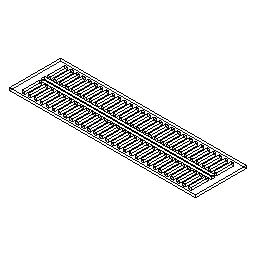
shelf small v2 (Autodesk Fusion 360 design; units mm, degrees)
Autodesk Fusion 360 part; units mm, degrees
sketch "Sketch1" plane through (0, 0, 0) normal (0, 0, 1) x (1, 0, 0)
  line L0 (109.5, -30) -> (-109.5, -30)
  line L1 (-109.5, -30) -> (-109.5, 30)
  line L2 (-109.5, 30) -> (109.5, 30)
  line L3 (109.5, 30) -> (109.5, -30)
  line L4 (109.5, -30) -> (-109.5, 30) construction
  line L5 (-109.5, -30) -> (109.5, 30) construction
  dimension "d1" = 60
  dimension "d2" = 219
  constraint horizontal L0
  constraint perpendicular L0 L1
  constraint parallel L0 L2
  constraint parallel L1 L3
  constraint coincident L4 origin
  constraint coincident L5 origin
  measures "d1" distance of L0.end L1.end
  measures "d2" distance of L1.end L2.end
extrude "Extrude1" add sketch "Sketch1" along normal blind 3
sketch "Sketch2" plane through (0, 0, 3) normal (0, 0, 1) x (-1, 0, 0)
  line L0 (-109.5, -30) -> (109.5, -30)
  line L1 (109.5, -30) -> (109.5, 30)
  line L2 (109.5, 30) -> (-109.5, 30)
  line L3 (-109.5, 30) -> (-109.5, -30)
  line L4 (-100, 2) -> (100, 2)
  line L5 (100, 2) -> (100, -2)
  line L6 (100, -2) -> (-100, -2)
  line L7 (-100, -2) -> (-100, 2)
  line L8 (-100, 2) -> (100, -2) construction
  line L9 (100, 2) -> (-100, -2) construction
  line L10 (36.5, -25) -> (33.5, -25)
  line L11 (33.5, -25) -> (33.5, -5)
  line L12 (33.5, -5) -> (36.5, -5)
  line L13 (36.5, -5) -> (36.5, -25)
  line L14 (29.5, -25) -> (26.5, -25)
  line L15 (26.5, -25) -> (26.5, -5)
  line L16 (26.5, -5) -> (29.5, -5)
  line L17 (29.5, -5) -> (29.5, -25)
  line L18 (22.5, -25) -> (19.5, -25)
  line L19 (19.5, -25) -> (19.5, -5)
  line L20 (19.5, -5) -> (22.5, -5)
  line L21 (22.5, -5) -> (22.5, -25)
  line L22 (15.5, -25) -> (12.5, -25)
  line L23 (12.5, -25) -> (12.5, -5)
  line L24 (12.5, -5) -> (15.5, -5)
  line L25 (15.5, -5) -> (15.5, -25)
  line L26 (8.5, -25) -> (5.5, -25)
  line L27 (5.5, -25) -> (5.5, -5)
  line L28 (5.5, -5) -> (8.5, -5)
  line L29 (8.5, -5) -> (8.5, -25)
  line L30 (1.5, -25) -> (-1.5, -25)
  line L31 (-1.5, -25) -> (-1.5, -5)
  line L32 (-1.5, -5) -> (1.5, -5)
  line L33 (1.5, -5) -> (1.5, -25)
  line L34 (-5.5, -25) -> (-8.5, -25)
  line L35 (-8.5, -25) -> (-8.5, -5)
  line L36 (-8.5, -5) -> (-5.5, -5)
  line L37 (-5.5, -5) -> (-5.5, -25)
  line L38 (-12.5, -25) -> (-15.5, -25)
  line L39 (-15.5, -25) -> (-15.5, -5)
  line L40 (-15.5, -5) -> (-12.5, -5)
  line L41 (-12.5, -5) -> (-12.5, -25)
  line L42 (-19.5, -25) -> (-22.5, -25)
  line L43 (-22.5, -25) -> (-22.5, -5)
  line L44 (-22.5, -5) -> (-19.5, -5)
  line L45 (-19.5, -5) -> (-19.5, -25)
  line L46 (-26.5, -25) -> (-29.5, -25)
  line L47 (-29.5, -25) -> (-29.5, -5)
  line L48 (-29.5, -5) -> (-26.5, -5)
  line L49 (-26.5, -5) -> (-26.5, -25)
  line L50 (-33.5, -25) -> (-36.5, -25)
  line L51 (-36.5, -25) -> (-36.5, -5)
  line L52 (-36.5, -5) -> (-33.5, -5)
  line L53 (-33.5, -5) -> (-33.5, -25)
  line L54 (-40.5, -25) -> (-43.5, -25)
  line L55 (-43.5, -25) -> (-43.5, -5)
  line L56 (-43.5, -5) -> (-40.5, -5)
  line L57 (-40.5, -5) -> (-40.5, -25)
  line L58 (-47.5, -25) -> (-50.5, -25)
  line L59 (-50.5, -25) -> (-50.5, -5)
  line L60 (-50.5, -5) -> (-47.5, -5)
  line L61 (-47.5, -5) -> (-47.5, -25)
  line L62 (-54.5, -25) -> (-57.5, -25)
  line L63 (-57.5, -25) -> (-57.5, -5)
  line L64 (-57.5, -5) -> (-54.5, -5)
  line L65 (-54.5, -5) -> (-54.5, -25)
  line L66 (-61.5, -25) -> (-64.5, -25)
  line L67 (-64.5, -25) -> (-64.5, -5)
  line L68 (-64.5, -5) -> (-61.5, -5)
  line L69 (-61.5, -5) -> (-61.5, -25)
  line L70 (-68.5, -25) -> (-71.5, -25)
  line L71 (-71.5, -25) -> (-71.5, -5)
  line L72 (-71.5, -5) -> (-68.5, -5)
  line L73 (-68.5, -5) -> (-68.5, -25)
  line L74 (-75.5, -5) -> (-78.5, -5)
  line L75 (-78.5, -5) -> (-78.5, -25)
  line L76 (-78.5, -25) -> (-75.5, -25)
  line L77 (-75.5, -25) -> (-75.5, -5)
  line L78 (-82.5, -5) -> (-85.5, -5)
  line L79 (-85.5, -5) -> (-85.5, -25)
  line L80 (-85.5, -25) -> (-82.5, -25)
  line L81 (-82.5, -25) -> (-82.5, -5)
  line L82 (-89.5, -5) -> (-92.5, -5)
  line L83 (-92.5, -5) -> (-92.5, -25)
  line L84 (-92.5, -25) -> (-89.5, -25)
  line L85 (-89.5, -25) -> (-89.5, -5)
  line L86 (-96.5, -5) -> (-99.5, -5)
  line L87 (-99.5, -5) -> (-99.5, -25)
  line L88 (-99.5, -25) -> (-96.5, -25)
  line L89 (-96.5, -25) -> (-96.5, -5)
  line L90 (36.5, 5) -> (33.5, 5)
  line L91 (33.5, 5) -> (33.5, 25)
  line L92 (33.5, 25) -> (36.5, 25)
  line L93 (36.5, 25) -> (36.5, 5)
  line L94 (29.5, 5) -> (26.5, 5)
  line L95 (26.5, 5) -> (26.5, 25)
  line L96 (26.5, 25) -> (29.5, 25)
  line L97 (29.5, 25) -> (29.5, 5)
  line L98 (22.5, 5) -> (19.5, 5)
  line L99 (19.5, 5) -> (19.5, 25)
  line L100 (19.5, 25) -> (22.5, 25)
  line L101 (22.5, 25) -> (22.5, 5)
  line L102 (15.5, 5) -> (12.5, 5)
  line L103 (12.5, 5) -> (12.5, 25)
  line L104 (12.5, 25) -> (15.5, 25)
  line L105 (15.5, 25) -> (15.5, 5)
  line L106 (8.5, 5) -> (5.5, 5)
  line L107 (5.5, 5) -> (5.5, 25)
  line L108 (5.5, 25) -> (8.5, 25)
  line L109 (8.5, 25) -> (8.5, 5)
  line L110 (1.5, 5) -> (-1.5, 5)
  line L111 (-1.5, 5) -> (-1.5, 25)
  line L112 (-1.5, 25) -> (1.5, 25)
  line L113 (1.5, 25) -> (1.5, 5)
  line L114 (-5.5, 5) -> (-8.5, 5)
  line L115 (-8.5, 5) -> (-8.5, 25)
  line L116 (-8.5, 25) -> (-5.5, 25)
  line L117 (-5.5, 25) -> (-5.5, 5)
  line L118 (-12.5, 5) -> (-15.5, 5)
  line L119 (-15.5, 5) -> (-15.5, 25)
  line L120 (-15.5, 25) -> (-12.5, 25)
  line L121 (-12.5, 25) -> (-12.5, 5)
  line L122 (-19.5, 5) -> (-22.5, 5)
  line L123 (-22.5, 5) -> (-22.5, 25)
  line L124 (-22.5, 25) -> (-19.5, 25)
  line L125 (-19.5, 25) -> (-19.5, 5)
  line L126 (-26.5, 5) -> (-29.5, 5)
  line L127 (-29.5, 5) -> (-29.5, 25)
  line L128 (-29.5, 25) -> (-26.5, 25)
  line L129 (-26.5, 25) -> (-26.5, 5)
  line L130 (-33.5, 5) -> (-36.5, 5)
  line L131 (-36.5, 5) -> (-36.5, 25)
  line L132 (-36.5, 25) -> (-33.5, 25)
  line L133 (-33.5, 25) -> (-33.5, 5)
  line L134 (-40.5, 5) -> (-43.5, 5)
  line L135 (-43.5, 5) -> (-43.5, 25)
  line L136 (-43.5, 25) -> (-40.5, 25)
  line L137 (-40.5, 25) -> (-40.5, 5)
  line L138 (-47.5, 5) -> (-50.5, 5)
  line L139 (-50.5, 5) -> (-50.5, 25)
  line L140 (-50.5, 25) -> (-47.5, 25)
  line L141 (-47.5, 25) -> (-47.5, 5)
  line L142 (-54.5, 5) -> (-57.5, 5)
  line L143 (-57.5, 5) -> (-57.5, 25)
  line L144 (-57.5, 25) -> (-54.5, 25)
  line L145 (-54.5, 25) -> (-54.5, 5)
  line L146 (-61.5, 5) -> (-64.5, 5)
  line L147 (-64.5, 5) -> (-64.5, 25)
  line L148 (-64.5, 25) -> (-61.5, 25)
  line L149 (-61.5, 25) -> (-61.5, 5)
  line L150 (-68.5, 5) -> (-71.5, 5)
  line L151 (-71.5, 5) -> (-71.5, 25)
  line L152 (-71.5, 25) -> (-68.5, 25)
  line L153 (-68.5, 25) -> (-68.5, 5)
  line L154 (-75.5, 5) -> (-78.5, 5)
  line L155 (-78.5, 5) -> (-78.5, 25)
  line L156 (-78.5, 25) -> (-75.5, 25)
  line L157 (-75.5, 25) -> (-75.5, 5)
  line L158 (-82.5, 5) -> (-85.5, 5)
  line L159 (-85.5, 5) -> (-85.5, 25)
  line L160 (-85.5, 25) -> (-82.5, 25)
  line L161 (-82.5, 25) -> (-82.5, 5)
  line L162 (-89.5, 5) -> (-92.5, 5)
  line L163 (-92.5, 5) -> (-92.5, 25)
  line L164 (-92.5, 25) -> (-89.5, 25)
  line L165 (-89.5, 25) -> (-89.5, 5)
  line L166 (-96.5, 5) -> (-99.5, 5)
  line L167 (-99.5, 5) -> (-99.5, 25)
  line L168 (-99.5, 25) -> (-96.5, 25)
  line L169 (-96.5, 25) -> (-96.5, 5)
  dimension "d5" = 200
  dimension "d6" = 4
  dimension "d7" = 3
  dimension "d8" = 3
  dimension "d9" = 3
  dimension "d10" = 3
  dimension "d11" = 3
  dimension "d12" = 3
  dimension "d13" = 3
  dimension "d14" = 4
  dimension "d15" = 4
  dimension "d16" = 4
  dimension "d17" = 4
  dimension "d18" = 4
  dimension "d19" = 4
  dimension "d20" = 4
  dimension "d21" = 4
  dimension "d22" = 4
  dimension "d23" = 4
  dimension "d24" = 4
  dimension "d25" = 4
  dimension "d26" = 4
  dimension "d27" = 4
  dimension "d28" = 4
  dimension "d29" = 4
  dimension "d30" = 4
  dimension "d31" = 4
  dimension "d32" = 4
  dimension "d33" = 3
  dimension "d34" = 3
  dimension "d35" = 3
  dimension "d36" = 3
  dimension "d37" = 3
  dimension "d38" = 3
  dimension "d39" = 3
  dimension "d40" = 3
  dimension "d42" = 3
  dimension "d43" = 3
  dimension "d44" = 3
  dimension "d45" = 3
  dimension "d46" = 3
  dimension "d47" = 3
  dimension "d48" = 3
  dimension "d49" = 3
  dimension "d50" = 3
  dimension "d51" = 3
  dimension "d52" = 3
  dimension "d53" = 3
  dimension "d54" = 3
  dimension "d55" = 3
  dimension "d56" = 3
  dimension "d57" = 3
  dimension "d58" = 3
  dimension "d59" = 3
  dimension "d60" = 3
  dimension "d61" = 3
  dimension "d62" = 3
  dimension "d63" = 3
  dimension "d64" = 3
  dimension "d65" = 3
  dimension "d66" = 3
  dimension "d67" = 4
  dimension "d68" = 4
  dimension "d69" = 4
  dimension "d70" = 4
  dimension "d71" = 4
  dimension "d72" = 4
  dimension "d73" = 4
  dimension "d74" = 4
  dimension "d75" = 4
  dimension "d76" = 4
  dimension "d77" = 4
  dimension "d78" = 4
  dimension "d79" = 4
  dimension "d80" = 4
  dimension "d81" = 4
  dimension "d82" = 4
  dimension "d83" = 4
  dimension "d84" = 4
  dimension "d85" = 4
  dimension "d86" = 10
  dimension "d87" = 10
  constraint horizontal L4
  constraint perpendicular L4 L5
  constraint parallel L4 L6
  constraint parallel L5 L7
  constraint coincident L8 origin
  constraint coincident L9 origin
  constraint horizontal L10
  constraint vertical L11
  constraint horizontal L12
  constraint vertical L13
  constraint horizontal L14
  constraint vertical L15
  constraint horizontal L16
  constraint vertical L17
  constraint horizontal L18
  constraint vertical L19
  constraint horizontal L20
  constraint vertical L21
  constraint horizontal L22
  constraint vertical L23
  constraint horizontal L24
  constraint vertical L25
  constraint horizontal L26
  constraint vertical L27
  constraint horizontal L28
  constraint vertical L29
  constraint horizontal L30
  constraint vertical L31
  constraint horizontal L32
  constraint vertical L33
  constraint horizontal L34
  constraint vertical L35
  constraint horizontal L36
  constraint vertical L37
  constraint horizontal L38
  constraint vertical L39
  constraint horizontal L40
  constraint vertical L41
  constraint horizontal L42
  constraint vertical L43
  constraint horizontal L44
  constraint vertical L45
  constraint horizontal L46
  constraint vertical L47
  constraint horizontal L48
  constraint vertical L49
  constraint horizontal L50
  constraint vertical L51
  constraint horizontal L52
  constraint vertical L53
  constraint horizontal L54
  constraint vertical L55
  constraint horizontal L56
  constraint vertical L57
  constraint horizontal L58
  constraint vertical L59
  constraint horizontal L60
  constraint vertical L61
  constraint horizontal L62
  constraint vertical L63
  constraint horizontal L64
  constraint vertical L65
  constraint horizontal L66
  constraint vertical L67
  constraint horizontal L68
  constraint vertical L69
  constraint horizontal L70
  constraint vertical L71
  constraint horizontal L72
  constraint vertical L73
  constraint horizontal L74
  constraint vertical L75
  constraint horizontal L76
  constraint vertical L77
  constraint horizontal L78
  constraint vertical L79
  constraint horizontal L80
  constraint vertical L81
  constraint horizontal L82
  constraint vertical L83
  constraint horizontal L84
  constraint vertical L85
  constraint horizontal L86
  constraint vertical L87
  constraint horizontal L88
  constraint vertical L89
  constraint horizontal L90
  constraint vertical L91
  constraint horizontal L92
  constraint vertical L93
  constraint horizontal L94
  constraint vertical L95
  constraint horizontal L96
  constraint vertical L97
  constraint horizontal L98
  constraint vertical L99
  constraint horizontal L100
  constraint vertical L101
  constraint horizontal L102
  constraint vertical L103
  constraint horizontal L104
  constraint vertical L105
  constraint horizontal L106
  constraint vertical L107
  constraint horizontal L108
  constraint vertical L109
  constraint horizontal L110
  constraint vertical L111
  constraint horizontal L112
  constraint vertical L113
  constraint horizontal L114
  constraint vertical L115
  constraint horizontal L116
  constraint vertical L117
  constraint horizontal L118
  constraint vertical L119
  constraint horizontal L120
  constraint vertical L121
  constraint horizontal L122
  constraint vertical L123
  constraint horizontal L124
  constraint vertical L125
  constraint horizontal L126
  constraint vertical L127
  constraint horizontal L128
  constraint vertical L129
  constraint horizontal L130
  constraint vertical L131
  constraint horizontal L132
  constraint vertical L133
  constraint horizontal L134
  constraint vertical L135
  constraint horizontal L136
  constraint vertical L137
  constraint horizontal L138
  constraint vertical L139
  constraint horizontal L140
  constraint vertical L141
  constraint horizontal L142
  constraint vertical L143
  constraint horizontal L144
  constraint vertical L145
  constraint horizontal L146
  constraint vertical L147
  constraint horizontal L148
  constraint vertical L149
  constraint horizontal L150
  constraint vertical L151
  constraint horizontal L152
  constraint vertical L153
  constraint horizontal L154
  constraint vertical L155
  constraint horizontal L156
  constraint vertical L157
  constraint horizontal L158
  constraint vertical L159
  constraint horizontal L160
  constraint vertical L161
  constraint horizontal L162
  constraint vertical L163
  constraint horizontal L164
  constraint vertical L165
  constraint horizontal L166
  constraint vertical L167
  constraint horizontal L168
  constraint vertical L169
  measures "d5" distance of L5.end L6.end
  measures "d6" distance of L4.end L5.end
  measures "d7" distance of L10.start L10.end
  measures "d8" distance of L14.start L14.end
  measures "d9" distance of L18.start L18.end
  measures "d10" distance of L22.start L22.end
  measures "d11" distance of L26.start L26.end
  measures "d12" distance of L30.start L30.end
  measures "d13" distance of L34.start L34.end
  measures "d14" distance of L11 L17
  measures "d15" distance of L15 L21
  measures "d16" distance of L19 L25
  measures "d17" distance of L23 L29
  measures "d18" distance of L27 L33
  measures "d19" distance of L31 L37
  measures "d20" distance of L35 L41
  measures "d21" distance of L39 L45
  measures "d22" distance of L43 L49
  measures "d23" distance of L47 L53
  measures "d24" distance of L51 L57
  measures "d25" distance of L55 L61
  measures "d26" distance of L59 L65
  measures "d27" distance of L63 L69
  measures "d28" distance of L67 L73
  measures "d29" distance of L71 L77
  measures "d30" distance of L75 L81
  measures "d31" distance of L79 L85
  measures "d32" distance of L83 L89
  measures "d33" distance of L38.start L38.end
  measures "d34" distance of L42.start L42.end
  measures "d35" distance of L46.start L46.end
  measures "d36" distance of L50.start L50.end
  measures "d37" distance of L54.start L54.end
  measures "d38" distance of L58.start L58.end
  measures "d39" distance of L62.start L62.end
  measures "d40" distance of L66.start L66.end
  measures "d42" distance of L70.start L70.end
  measures "d43" distance of L75.end L76.end
  measures "d44" distance of L79.end L80.end
  measures "d45" distance of L83.end L84.end
  measures "d46" distance of L87.end L88.end
  measures "d47" distance of L91.end L92.end
  measures "d48" distance of L95.end L96.end
  measures "d49" distance of L99.end L100.end
  measures "d50" distance of L103.end L104.end
  measures "d51" distance of L107.end L108.end
  measures "d52" distance of L111.end L112.end
  measures "d53" distance of L115.end L116.end
  measures "d54" distance of L119.end L120.end
  measures "d55" distance of L123.end L124.end
  measures "d56" distance of L127.end L128.end
  measures "d57" distance of L131.end L132.end
  measures "d58" distance of L135.end L136.end
  measures "d59" distance of L139.end L140.end
  measures "d60" distance of L143.end L144.end
  measures "d61" distance of L147.end L148.end
  measures "d62" distance of L151.end L152.end
  measures "d63" distance of L155.end L156.end
  measures "d64" distance of L159.end L160.end
  measures "d65" distance of L163.end L164.end
  measures "d66" distance of L167.end L168.end
  measures "d67" distance of L163 L169
  measures "d68" distance of L159 L165
  measures "d69" distance of L155 L161
  measures "d70" distance of L151 L157
  measures "d71" distance of L147 L153
  measures "d72" distance of L143 L149
  measures "d73" distance of L139 L145
  measures "d74" distance of L135 L141
  measures "d75" distance of L131 L137
  measures "d76" distance of L127 L133
  measures "d77" distance of L123 L129
  measures "d78" distance of L119 L125
  measures "d79" distance of L115 L121
  measures "d80" distance of L111 L117
  measures "d81" distance of L107 L113
  measures "d82" distance of L103 L109
  measures "d83" distance of L99 L105
  measures "d84" distance of L95 L101
  measures "d85" distance of L91 L97
  measures "d86" distance of L3 L87
  measures "d87" distance of L3 L167
sketch "Sketch3" plane through (0, 0, 3) normal (0, 0, 1) x (-1, 0, 0)
  line L0 (40.5, -25) -> (43.5, -25)
  line L1 (43.5, -25) -> (43.5, -5)
  line L2 (43.5, -5) -> (40.5, -5)
  line L3 (40.5, -5) -> (40.5, -25)
  line L4 (47.5, -25) -> (50.5, -25)
  line L5 (50.5, -25) -> (50.5, -5)
  line L6 (50.5, -5) -> (47.5, -5)
  line L7 (47.5, -5) -> (47.5, -25)
  line L8 (54.5, -25) -> (57.5, -25)
  line L9 (57.5, -25) -> (57.5, -5)
  line L10 (57.5, -5) -> (54.5, -5)
  line L11 (54.5, -5) -> (54.5, -25)
  line L12 (61.5, -25) -> (64.5, -25)
  line L13 (64.5, -25) -> (64.5, -5)
  line L14 (64.5, -5) -> (61.5, -5)
  line L15 (61.5, -5) -> (61.5, -25)
  line L16 (68.5, -25) -> (71.5, -25)
  line L17 (71.5, -25) -> (71.5, -5)
  line L18 (71.5, -5) -> (68.5, -5)
  line L19 (68.5, -5) -> (68.5, -25)
  line L20 (75.5, -25) -> (78.5, -25)
  line L21 (78.5, -25) -> (78.5, -5)
  line L22 (78.5, -5) -> (75.5, -5)
  line L23 (75.5, -5) -> (75.5, -25)
  line L24 (82.5, -25) -> (85.5, -25)
  line L25 (85.5, -25) -> (85.5, -5)
  line L26 (85.5, -5) -> (82.5, -5)
  line L27 (82.5, -5) -> (82.5, -25)
  line L28 (85.5, 5) -> (82.5, 5)
  line L29 (82.5, 5) -> (82.5, 25)
  line L30 (82.5, 25) -> (85.5, 25)
  line L31 (85.5, 25) -> (85.5, 5)
  line L32 (78.5, 5) -> (75.5, 5)
  line L33 (75.5, 5) -> (75.5, 25)
  line L34 (75.5, 25) -> (78.5, 25)
  line L35 (78.5, 25) -> (78.5, 5)
  line L36 (71.5, 5) -> (68.5, 5)
  line L37 (68.5, 5) -> (68.5, 25)
  line L38 (68.5, 25) -> (71.5, 25)
  line L39 (71.5, 25) -> (71.5, 5)
  line L40 (64.5, 5) -> (61.5, 5)
  line L41 (61.5, 5) -> (61.5, 25)
  line L42 (61.5, 25) -> (64.5, 25)
  line L43 (64.5, 25) -> (64.5, 5)
  line L44 (57.5, 5) -> (54.5, 5)
  line L45 (54.5, 5) -> (54.5, 25)
  line L46 (54.5, 25) -> (57.5, 25)
  line L47 (57.5, 25) -> (57.5, 5)
  line L48 (50.5, 5) -> (47.5, 5)
  line L49 (47.5, 5) -> (47.5, 25)
  line L50 (47.5, 25) -> (50.5, 25)
  line L51 (50.5, 25) -> (50.5, 5)
  line L52 (43.5, 5) -> (40.5, 5)
  line L53 (40.5, 5) -> (40.5, 25)
  line L54 (40.5, 25) -> (43.5, 25)
  line L55 (43.5, 25) -> (43.5, 5)
  line L56 (36.5, -5) -> (36.5, -25)
  line L57 (36.5, 25) -> (36.5, 5)
  line L58 (89.5, -25) -> (92.5, -25)
  line L59 (92.5, -25) -> (92.5, -5)
  line L60 (92.5, -5) -> (89.5, -5)
  line L61 (89.5, -5) -> (89.5, -25)
  line L62 (89.5, 5) -> (92.5, 5)
  line L63 (92.5, 5) -> (92.5, 25)
  line L64 (92.5, 25) -> (89.5, 25)
  line L65 (89.5, 25) -> (89.5, 5)
  line L66 (96.5, 5) -> (99.5, 5)
  line L67 (99.5, 5) -> (99.5, 25)
  line L68 (99.5, 25) -> (96.5, 25)
  line L69 (96.5, 25) -> (96.5, 5)
  line L70 (96.5, -5) -> (99.5, -5)
  line L71 (99.5, -5) -> (99.5, -25)
  line L72 (99.5, -25) -> (96.5, -25)
  line L73 (96.5, -25) -> (96.5, -5)
  dimension "d88" = 4
  dimension "d89" = 4
  dimension "d90" = 4
  dimension "d91" = 4
  dimension "d92" = 4
  dimension "d93" = 4
  dimension "d94" = 4
  dimension "d95" = 4
  dimension "d96" = 4
  dimension "d97" = 4
  dimension "d98" = 4
  dimension "d99" = 4
  dimension "d100" = 4
  dimension "d101" = 4
  dimension "d102" = 3
  dimension "d103" = 3
  dimension "d104" = 3
  dimension "d105" = 3
  dimension "d106" = 3
  dimension "d107" = 3
  dimension "d108" = 3
  dimension "d109" = 3
  dimension "d110" = 3
  dimension "d111" = 3
  dimension "d112" = 3
  dimension "d113" = 3
  dimension "d114" = 3
  dimension "d115" = 3
  dimension "d116" = 4
  dimension "d117" = 3
  dimension "d118" = 4
  dimension "d119" = 3
  dimension "d120" = 4
  dimension "d121" = 4
  dimension "d122" = 3
  dimension "d123" = 3
  constraint horizontal L0
  constraint vertical L1
  constraint horizontal L2
  constraint vertical L3
  constraint horizontal L4
  constraint vertical L5
  constraint horizontal L6
  constraint vertical L7
  constraint horizontal L8
  constraint vertical L9
  constraint horizontal L10
  constraint vertical L11
  constraint horizontal L12
  constraint vertical L13
  constraint horizontal L14
  constraint vertical L15
  constraint horizontal L16
  constraint vertical L17
  constraint horizontal L18
  constraint vertical L19
  constraint horizontal L20
  constraint vertical L21
  constraint horizontal L22
  constraint vertical L23
  constraint horizontal L24
  constraint vertical L25
  constraint horizontal L26
  constraint vertical L27
  constraint horizontal L28
  constraint vertical L29
  constraint horizontal L30
  constraint vertical L31
  constraint horizontal L32
  constraint vertical L33
  constraint horizontal L34
  constraint vertical L35
  constraint horizontal L36
  constraint vertical L37
  constraint horizontal L38
  constraint vertical L39
  constraint horizontal L40
  constraint vertical L41
  constraint horizontal L42
  constraint vertical L43
  constraint horizontal L44
  constraint vertical L45
  constraint horizontal L46
  constraint vertical L47
  constraint horizontal L48
  constraint vertical L49
  constraint horizontal L50
  constraint vertical L51
  constraint horizontal L52
  constraint vertical L53
  constraint horizontal L54
  constraint vertical L55
  constraint horizontal L58
  constraint vertical L59
  constraint horizontal L60
  constraint vertical L61
  constraint horizontal L62
  constraint vertical L63
  constraint horizontal L64
  constraint vertical L65
  constraint horizontal L66
  constraint vertical L67
  constraint horizontal L68
  constraint vertical L69
  constraint horizontal L70
  constraint vertical L71
  constraint horizontal L72
  constraint vertical L73
  measures "d88" distance of L3 L56
  measures "d89" distance of L1 L7
  measures "d90" distance of L5 L11
  measures "d91" distance of L9 L15
  measures "d92" distance of L13 L19
  measures "d93" distance of L17 L23
  measures "d94" distance of L21 L27
  measures "d95" distance of L49 L55
  measures "d96" distance of L45 L51
  measures "d97" distance of L41 L47
  measures "d98" distance of L37 L43
  measures "d99" distance of L33 L39
  measures "d100" distance of L29 L35
  measures "d101" distance of L53 L57
  measures "d102" distance of L24.start L24.end
  measures "d103" distance of L20.start L20.end
  measures "d104" distance of L16.start L16.end
  measures "d105" distance of L12.start L12.end
  measures "d106" distance of L8.start L8.end
  measures "d107" distance of L4.start L4.end
  measures "d108" distance of L0.start L0.end
  measures "d109" distance of L53.end L54.end
  measures "d110" distance of L49.end L50.end
  measures "d111" distance of L45.end L46.end
  measures "d112" distance of L41.end L42.end
  measures "d113" distance of L37.end L38.end
  measures "d114" distance of L33.end L34.end
  measures "d115" distance of L29.end L30.end
  measures "d116" distance of L25 L61
  measures "d117" distance of L58.start L58.end
  measures "d118" distance of L59 L73
  measures "d119" distance of L71.end L72.end
  measures "d120" distance of L31 L65
  measures "d121" distance of L63 L69
  measures "d122" distance of L63.end L64.end
  measures "d123" distance of L67.end L68.end
extrude "Extrude2" cut sketch "Sketch2" against normal blind 5 contours L4 L5 L6 L7 | L10 L11 L12 L13 | L14 L15 L16 L17 | L18 L19 L20 L21 | L22 L23 L24 L25 | L26 L27 L28 L29 | L30 L31 L32 L33 | L34 L35 L36 L37 | L38 L39 L40 L41 | L42 L43 L44 L45 | L46 L47 L48 L49 | L50 L51 L52 L53 | L54 L55 L56 L57 | L58 L59 L60 L61 | L62 L63 L64 L65 | L66 L67 L68 L69 | L70 L71 L72 L73 | L74 L75 L76 L77 | L78 L79 L80 L81 | L82 L83 L84 L85 | L86 L87 L88 L89 | L90 L91 L92 L93 | L94 L95 L96 L97 | L98 L99 L100 L101 | L102 L103 L104 L105 | L106 L107 L108 L109 | L110 L111 L112 L113 | L114 L115 L116 L117 | L118 L119 L120 L121 | L122 L123 L124 L125 | L126 L127 L128 L129 | L130 L131 L132 L133 | L134 L135 L136 L137 | L138 L139 L140 L141 | L142 L143 L144 L145 | L146 L147 L148 L149 | L150 L151 L152 L153 | L154 L155 L156 L157 | L158 L159 L160 L161 | L162 L163 L164 L165 | L166 L167 L168 L169
extrude "Extrude3" cut sketch "Sketch3" against normal blind 5
